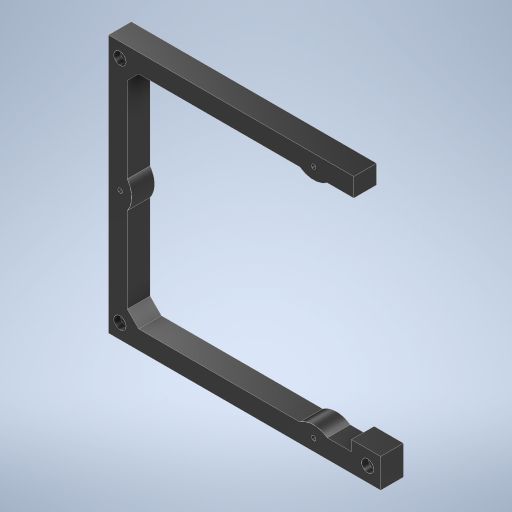
# Autodesk Inventor part: display_cover_part2
Saved by Autodesk Inventor 2024.3 (Build 283343000, 343)
## iProperties
Created: 2024-12-14
Part Number: display_cover_part2
Material: Polystyren
Document SubType Name: Modeling
Designer: Marek
Density: 1.021 g/cm^3
Appearance: Lesklá – černá
Author: Marek
Autodesk Inventor part; units mm, degrees
ref_plane "YZ Plane" through (0, 0, 0) normal (1, 0, 0) x (0, 1, 0)
ref_plane "XZ Plane" through (0, 0, 0) normal (0, 1, 0) x (-1, 0, 0)
ref_plane "XY Plane" through (0, 0, 0) normal (0, 0, 1) x (1, 0, 0)
sketch "Náčrt1" plane through (0, 0, 0) normal (0, 0, 1) x (1, 0, 0)
  line L0 (0, 110.95) -> (0, -110.95) projected
  line L1 (-116.9, 0) -> (116.9, 0) projected
  line L2 (67, 79.25) -> (-83.5, 79.25)
  line L3 (-83.5, 79.25) -> (-83.5, -79.25)
  line L4 (-83.5, -79.25) -> (83.5, -79.25)
  line L5 (83.5, -79.25) -> (83.5, -61.25)
  line L6 (83.5, -61.25) -> (65.5, -61.25)
  line L7 (65.5, -61.25) -> (65.5, -67.75)
  line L8 (65.5, -67.75) -> (-72, -67.75)
  line L9 (-72, -67.75) -> (-72, 67.75)
  line L10 (-72, 67.75) -> (67, 67.75)
  line L11 (67, 67.75) -> (67, 79.25)
  arc A0 (-72, -8.415) -> (-72, 8.415) centre (-83.5, 0) ccw
  arc A1 (33.935, 67.75) -> (50.765, 67.75) centre (42.35, 79.25) ccw
  arc A2 (50.765, -67.75) -> (33.935, -67.75) centre (42.35, -79.25) ccw
  point P0 (0, 0)
  dimension "d0" = 11.5
  dimension "d1" = 11.5
  dimension "d2" = 11.5
  dimension "d3" = 150.5
  dimension "d4" = 158.5
  dimension "d5" = 167
  dimension "d6" = 18
  dimension "d7" = 18
  dimension "d8" = 83.5
  dimension "d32" = 28.5
  dimension "d33" = 28.5
  dimension "d35" = 42.35
  dimension "d36" = 42.35
  dimension "d37" = 14.25
  constraints: 20 end point, 9 perpendicular, 8 point on line, 6 point on circle, 3 centre point, 1 horizontal, 1 midpoint, 1 other
  measures "d0" distance between parallel lines of L10 L2
  measures "d1" distance between parallel lines of L3 L9
  measures "d2" distance between parallel lines of L4 L8
  measures "d3" distance between parallel lines of L3 L11
  measures "d4" distance between parallel lines of L4 L2
  measures "d5" distance between parallel lines of L3 L5
  measures "d6" distance between parallel lines of L5 L7
  measures "d7" distance between parallel lines of L4 L6
  measures "d8" distance between parallel lines of L0 L3
  measures "d32" diameter of A0
  measures "d33" diameter of A1
  measures "d35" distance from line of A1.centre L0
  measures "d36" distance from line of A2.centre L0
  measures "d37" radius of A2
extrude "Vysunutí1" add sketch "Náčrt1" along normal blind 14 contours L2 L11 L10 L0 | L0 L10 L9 L1 L3 L2 | L10 A1 | L1 L9 L8 L0 L4 L3 | L8 L7 L6 L5 L4 L0 | A0 L9 L1 | L1 L9 A0 | A2 L8
chamfer "Zkosení1" distance 7 angle 45 2 edges at (-72, 67.75, 7) (-72, -67.75, 7)
sketch "Náčrt2" plane through (0, 0, 14) normal (0, 0, 1) x (1, 0, 0)
  line L0 (67, 79.25) -> (-83.5, 79.25) projected
  line L1 (-83.5, 79.25) -> (-83.5, -79.25) projected
  line L2 (-83.5, -79.25) -> (83.5, -79.25) projected
  line L3 (83.5, -79.25) -> (83.5, -61.25) projected
  line L4 (83.5, -61.25) -> (65.5, -61.25) projected
  line L5 (65.5, -61.25) -> (65.5, -67.75) projected
  line L6 (65.5, -67.75) -> (50.765, -67.75) projected
  line L7 (-72, -60.75) -> (-65, -67.75) projected
  line L8 (-72, -60.75) -> (-72, -8.415) projected
  line L9 (-65, 67.75) -> (-72, 60.75) projected
  line L10 (-65, 67.75) -> (33.935, 67.75) projected
  line L11 (67, 67.75) -> (67, 79.25) projected
  line L12 (0, 110.95) -> (0, -110.95) projected
  line L13 (-116.9, 0) -> (116.9, 0) projected
  circle A0 centre (-76.5, 70.25) radius 3.75
  circle A1 centre (-76.5, -70.25) radius 3.75
  circle A2 centre (75.5, -70.25) radius 3.75
  arc A3 (50.765, -67.75) -> (33.935, -67.75) centre (42.35, -79.25) ccw projected
  line L14 (33.935, -67.75) -> (-65, -67.75) projected
  arc A4 (-72, -8.415) -> (-72, 8.415) centre (-83.5, 0) ccw projected
  line L15 (-72, 8.415) -> (-72, 60.75) projected
  arc A5 (33.935, 67.75) -> (50.765, 67.75) centre (42.35, 79.25) ccw projected
  line L16 (50.765, 67.75) -> (67, 67.75) projected
  point P0 (0, 0)
  dimension "d14" = 7.5
  dimension "d15" = 7.5
  dimension "d16" = 7.5
  dimension "d17" = 9
  dimension "d18" = 9
  dimension "d19" = 9
  dimension "d20" = 7
  dimension "d21" = 7
  dimension "d22" = 8
  constraints: 3 centre point
  measures "d14" diameter of A0
  measures "d15" diameter of A1
  measures "d16" diameter of A2
  measures "d17" distance from line of L2 A1.centre
  measures "d18" distance from line of L2 A2.centre
  measures "d19" distance from line of L0 A0.centre
  measures "d20" distance from line of L1 A0.centre
  measures "d21" distance from line of L1 A1.centre
  measures "d22" distance from line of A2.centre L3
extrude "Vysunutí2" cut sketch "Náčrt2" against normal blind 4 contours A0 | A1 | A2
sketch "Náčrt3" plane through (-76.5, 70.25, 10) normal (0, 0, 1) x (1, 0, 0)
  circle A0 centre (0, 0) radius 3.75 projected
  circle A1 centre (0, -140.5) radius 3.75 projected
  circle A2 centre (152, -140.5) radius 3.75 projected
  circle A3 centre (0, 0) radius 3.75 projected
  point P0 (76.5, -70.25)
  constraints: 3 coincident
hole "Díra1" at (-76.5, 70.25, 10) at (-76.5, -70.25, 10) at (75.5, -70.25, 10) direction (0, 0, -1) diameter 3.7 end through all
sketch "Náčrt4" plane through (0, 0, 0) normal (0, 0, -1) x (-1, 0, 0)
  circle A0 centre (76.5, -70.25) radius 1.85 projected
  circle A1 centre (76.5, 70.25) radius 1.85 projected
  circle A2 centre (-75.5, -70.25) radius 1.85 projected
  line L0 (-67, 79.25) -> (83.5, 79.25) projected
  line L1 (-67, 67.75) -> (-67, 79.25) projected
  line L2 (-50.765, 67.75) -> (-67, 67.75) projected
  arc A3 (-50.765, 67.75) -> (-33.935, 67.75) centre (-42.35, 79.25) ccw projected
  line L3 (65, 67.75) -> (-33.935, 67.75) projected
  line L4 (72, 60.75) -> (65, 67.75) projected
  line L5 (72, 8.415) -> (72, 60.75) projected
  arc A4 (72, 8.415) -> (72, -8.415) centre (83.5, 0) ccw projected
  line L6 (72, -60.75) -> (72, -8.415) projected
  line L7 (65, -67.75) -> (72, -60.75) projected
  line L8 (-33.935, -67.75) -> (65, -67.75) projected
  arc A5 (-33.935, -67.75) -> (-50.765, -67.75) centre (-42.35, -79.25) ccw projected
  line L9 (-65.5, -67.75) -> (-50.765, -67.75) projected
  line L10 (-65.5, -61.25) -> (-65.5, -67.75) projected
  line L11 (-83.5, -61.25) -> (-65.5, -61.25) projected
  line L12 (-83.5, -79.25) -> (-83.5, -61.25) projected
  line L13 (83.5, -79.25) -> (-83.5, -79.25) projected
  line L14 (83.5, 79.25) -> (83.5, -79.25) projected
  line L15 (0, -110.95) -> (0, 110.95) projected
  line L16 (-116.9, 0) -> (116.9, 0) projected
  point P0 (0, 0)
  point P1 (34.5, 72.45)
  dimension "d38" = 49
  dimension "d39" = 6.8
  measures "d38" distance from line of L14 point (34.5, 72.45)
  measures "d39" distance from line of L0 point (34.5, 72.45)
hole "Díra2" at (-34.5, 72.45, 0) direction (0, 0, 1) diameter 5 depth 4.3
sketch "Náčrt5" plane through (0, 0, 14) normal (0, 0, 1) x (1, 0, 0)
  arc A0 (33.935, 67.75) -> (50.765, 67.75) centre (42.35, 79.25) ccw projected
  arc A1 (-72, -8.415) -> (-72, 8.415) centre (-83.5, 0) ccw projected
  arc A2 (50.765, -67.75) -> (33.935, -67.75) centre (42.35, -79.25) ccw projected
  line L0 (-116.9, 0) -> (116.9, 0) projected
  line L1 (0, 110.95) -> (0, -110.95) projected
  circle A3 centre (75.5, -70.25) radius 3.75 projected
  circle A4 centre (-76.5, -70.25) radius 3.75 projected
  circle A5 centre (-76.5, 70.25) radius 3.75 projected
  line L2 (67, 79.25) -> (-83.5, 79.25) projected
  line L3 (-83.5, 79.25) -> (-83.5, -79.25) projected
  line L4 (-83.5, -79.25) -> (83.5, -79.25) projected
  line L5 (83.5, -79.25) -> (83.5, -61.25) projected
  line L6 (83.5, -61.25) -> (65.5, -61.25) projected
  line L7 (65.5, -61.25) -> (65.5, -67.75) projected
  line L8 (65.5, -67.75) -> (50.765, -67.75) projected
  arc A6 (50.765, -67.75) -> (33.935, -67.75) centre (42.35, -79.25) ccw projected
  line L9 (33.935, -67.75) -> (-65, -67.75) projected
  line L10 (-72, -60.75) -> (-65, -67.75) projected
  line L11 (-72, -60.75) -> (-72, -8.415) projected
  arc A7 (-72, -8.415) -> (-72, 8.415) centre (-83.5, 0) ccw projected
  line L12 (-72, 8.415) -> (-72, 60.75) projected
  line L13 (-65, 67.75) -> (-72, 60.75) projected
  line L14 (-65, 67.75) -> (33.935, 67.75) projected
  arc A8 (33.935, 67.75) -> (50.765, 67.75) centre (42.35, 79.25) ccw projected
  line L15 (50.765, 67.75) -> (67, 67.75) projected
  line L16 (67, 67.75) -> (67, 79.25) projected
  point P0 (0, 0)
  point P1 (-76.375, 0)
  point P2 (42.35, 72.125)
  point P3 (42.35, -72.125)
  dimension "d47" = 7.125
  dimension "d48" = 42.35
  dimension "d49" = 7.125
  dimension "d50" = 42.35
  dimension "d51" = 7.125
  constraints: 1 point on line
  measures "d47" distance from line of point (42.35, -72.125) L4
  measures "d48" distance from line of L1 point (42.35, -72.125)
  measures "d49" distance from line of L2 point (42.35, 72.125)
  measures "d50" distance from line of L1 point (42.35, 72.125)
  measures "d51" distance from line of L3 point (-76.375, 0)
hole "Díra3" at (-76.375, 0, 14) at (42.35, 72.125, 14) at (42.35, -72.125, 14) direction (0, 0, -1) diameter 2.8 depth 14
equation "\"d49\" = d47"
equation "\"d51\" = d47"
